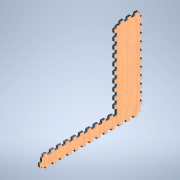
# Autodesk Inventor part: plate_side
Saved by Autodesk Inventor 2021 (Build 250183000, 183)
## iProperties
Created: 2021-03-07
Part Number: plate_side
Material: Generisch
Document SubType Name: Modeling
Designer: Tilman
Density: 1 g/cm^3
Appearance: Glänzend - Schwarz
Author: Tilman
Autodesk Inventor part; units mm, degrees
ref_plane "YZ Plane" through (0, 0, 0) normal (1, 0, 0) x (0, 1, 0)
ref_plane "XZ Plane" through (0, 0, 0) normal (0, 1, 0) x (-1, 0, 0)
ref_plane "XY Plane" through (0, 0, 0) normal (0, 0, 1) x (1, 0, 0)
sketch "Skizze1" plane through (0, 0, 0) normal (1, 0, 0) x (0, 1, 0)
  line L0 (5, 0) -> (5, -3)
  line L1 (5, -3) -> (3, -3)
  line L2 (3, -3) -> (3, -8)
  line L3 (3, -8) -> (0, -8)
  line L4 (0, -8) -> (0, -13)
  line L5 (0, -13) -> (3, -13)
  line L6 (3, -13) -> (3, -18)
  line L7 (3, -18) -> (0, -18)
  line L8 (0, -18) -> (0, -23)
  line L9 (0, -23) -> (3, -23)
  line L10 (3, -23) -> (3, -28)
  line L11 (3, -28) -> (0, -28)
  line L12 (0, -28) -> (0, -33)
  line L13 (0, -33) -> (3, -33)
  line L14 (3, -33) -> (3, -38)
  line L15 (3, -38) -> (0, -38)
  line L16 (0, -38) -> (0, -43)
  line L17 (0, -43) -> (3, -43)
  line L18 (3, -43) -> (3, -48)
  line L19 (3, -48) -> (0, -48)
  line L20 (0, -48) -> (0, -53)
  line L21 (0, -53) -> (3, -53)
  line L22 (3, -53) -> (3, -58)
  line L23 (3, -58) -> (0, -58)
  line L24 (0, -58) -> (0, -63)
  line L25 (0, -63) -> (3, -63)
  line L26 (3, -63) -> (3, -68)
  line L27 (3, -68) -> (0, -68)
  line L28 (0, -68) -> (0, -73)
  line L29 (0, -73) -> (3, -73)
  line L30 (3, -73) -> (3, -78)
  line L31 (3, -78) -> (0, -78)
  line L32 (0, -78) -> (0, -83)
  line L33 (0, -83) -> (3, -83)
  line L34 (3, -83) -> (3, -88)
  line L35 (3, -88) -> (0, -88)
  line L36 (0, -88) -> (0, -93)
  line L37 (0, -93) -> (3, -93)
  line L38 (3, -93) -> (3, -98)
  line L39 (3, -98) -> (0, -98)
  line L40 (0, -98) -> (0, -103)
  line L41 (0, -103) -> (3, -103)
  line L42 (3, -133) -> (3, -137)
  line L43 (3, -137) -> (10, -137)
  line L44 (10, -137) -> (10, -140)
  line L45 (10, -140) -> (15, -140)
  line L46 (15, -140) -> (15, -137)
  line L47 (15, -137) -> (20, -137)
  line L48 (25, -137) -> (30, -137)
  line L49 (25, -140) -> (25, -137)
  line L50 (20, -140) -> (25, -140)
  line L51 (20, -137) -> (20, -140)
  line L52 (35, -137) -> (40, -137)
  line L53 (35, -140) -> (35, -137)
  line L54 (30, -140) -> (35, -140)
  line L55 (30, -137) -> (30, -140)
  line L56 (45, -137) -> (50, -137)
  line L57 (45, -140) -> (45, -137)
  line L58 (40, -140) -> (45, -140)
  line L59 (40, -137) -> (40, -140)
  line L60 (55, -137) -> (60, -137)
  line L61 (55, -140) -> (55, -137)
  line L62 (50, -140) -> (55, -140)
  line L63 (50, -137) -> (50, -140)
  line L64 (65, -137) -> (70, -137)
  line L65 (65, -140) -> (65, -137)
  line L66 (60, -140) -> (65, -140)
  line L67 (60, -137) -> (60, -140)
  line L68 (75, -137) -> (80, -137)
  line L69 (75, -140) -> (75, -137)
  line L70 (70, -140) -> (75, -140)
  line L71 (70, -137) -> (70, -140)
  line L72 (85, -137) -> (90, -137)
  line L73 (85, -140) -> (85, -137)
  line L74 (80, -140) -> (85, -140)
  line L75 (80, -137) -> (80, -140)
  line L76 (95, -137) -> (100, -137)
  line L77 (95, -140) -> (95, -137)
  line L78 (90, -140) -> (95, -140)
  line L79 (90, -137) -> (90, -140)
  line L80 (105, -137) -> (110, -137)
  line L81 (105, -140) -> (105, -137)
  line L82 (100, -140) -> (105, -140)
  line L83 (100, -137) -> (100, -140)
  line L84 (115, -137) -> (120, -137)
  line L85 (115, -140) -> (115, -137)
  line L86 (110, -140) -> (115, -140)
  line L87 (110, -137) -> (110, -140)
  line L88 (120, -137) -> (120, -135)
  line L89 (120, -135) -> (123, -135)
  line L90 (123, -135) -> (123, -130)
  line L91 (123, -130) -> (120, -130)
  line L92 (120, -130) -> (120, -125)
  line L93 (120, -105) -> (118, -105)
  line L94 (118, -105) -> (118, -102)
  line L95 (118, -102) -> (113, -102)
  line L96 (113, -102) -> (113, -105)
  line L97 (113, -105) -> (108, -105)
  line L98 (103, -105) -> (98, -105)
  line L99 (103, -102) -> (103, -105)
  line L100 (108, -102) -> (103, -102)
  line L101 (108, -105) -> (108, -102)
  line L102 (93, -105) -> (88, -105)
  line L103 (93, -102) -> (93, -105)
  line L104 (98, -102) -> (93, -102)
  line L105 (98, -105) -> (98, -102)
  line L106 (83, -105) -> (78, -105)
  line L107 (83, -102) -> (83, -105)
  line L108 (88, -102) -> (83, -102)
  line L109 (88, -105) -> (88, -102)
  line L110 (73, -105) -> (68, -105)
  line L111 (73, -102) -> (73, -105)
  line L112 (78, -102) -> (73, -102)
  line L113 (78, -105) -> (78, -102)
  line L114 (63, -105) -> (58, -105)
  line L115 (63, -102) -> (63, -105)
  line L116 (68, -102) -> (63, -102)
  line L117 (68, -105) -> (68, -102)
  line L118 (53, -105) -> (48, -105)
  line L119 (53, -102) -> (53, -105)
  line L120 (58, -102) -> (53, -102)
  line L121 (58, -105) -> (58, -102)
  line L122 (43, -105) -> (38, -105)
  line L123 (43, -102) -> (43, -105)
  line L124 (48, -102) -> (43, -102)
  line L125 (48, -105) -> (48, -102)
  line L126 (33, -105) -> (28, -105)
  line L127 (33, -102) -> (33, -105)
  line L128 (38, -102) -> (33, -102)
  line L129 (38, -105) -> (38, -102)
  line L130 (23, -105) -> (18, -105)
  line L131 (23, -102) -> (23, -105)
  line L132 (28, -102) -> (23, -102)
  line L133 (28, -105) -> (28, -102)
  line L134 (5, 0) -> (10, 0)
  line L135 (10, 0) -> (10, -3)
  line L136 (10, -3) -> (15, -3)
  line L137 (18, -105) -> (15, -105)
  line L138 (15, -105) -> (15, -100)
  line L139 (15, -100) -> (18, -100)
  line L140 (18, -100) -> (18, -95)
  line L141 (18, -90) -> (18, -85)
  line L142 (18, -95) -> (15, -95)
  line L143 (15, -90) -> (18, -90)
  line L144 (15, -95) -> (15, -90)
  line L145 (18, -80) -> (18, -75)
  line L146 (18, -85) -> (15, -85)
  line L147 (15, -80) -> (18, -80)
  line L148 (15, -85) -> (15, -80)
  line L149 (18, -70) -> (18, -65)
  line L150 (18, -75) -> (15, -75)
  line L151 (15, -70) -> (18, -70)
  line L152 (15, -75) -> (15, -70)
  line L153 (18, -60) -> (18, -55)
  line L154 (18, -65) -> (15, -65)
  line L155 (15, -60) -> (18, -60)
  line L156 (15, -65) -> (15, -60)
  line L157 (18, -50) -> (18, -45)
  line L158 (18, -55) -> (15, -55)
  line L159 (15, -50) -> (18, -50)
  line L160 (15, -55) -> (15, -50)
  line L161 (18, -40) -> (18, -35)
  line L162 (18, -45) -> (15, -45)
  line L163 (15, -40) -> (18, -40)
  line L164 (15, -45) -> (15, -40)
  line L165 (18, -30) -> (18, -25)
  line L166 (18, -35) -> (15, -35)
  line L167 (15, -30) -> (18, -30)
  line L168 (15, -35) -> (15, -30)
  line L169 (3, -103) -> (3, -108)
  line L170 (3, -108) -> (0, -108)
  line L171 (0, -108) -> (0, -113)
  line L172 (0, -113) -> (3, -113)
  line L173 (3, -113) -> (3, -118)
  line L174 (3, -118) -> (0, -118)
  line L175 (0, -118) -> (0, -123)
  line L176 (0, -123) -> (3, -123)
  line L177 (18, -20) -> (18, -15)
  line L178 (18, -25) -> (15, -25)
  line L179 (15, -20) -> (18, -20)
  line L180 (15, -25) -> (15, -20)
  line L181 (18, -10) -> (18, -5)
  line L182 (18, -15) -> (15, -15)
  line L183 (15, -10) -> (18, -10)
  line L184 (15, -15) -> (15, -10)
  line L185 (15, -5) -> (18, -5)
  line L186 (3, -123) -> (3, -128)
  line L187 (3, -128) -> (0, -128)
  line L188 (0, -128) -> (0, -133)
  line L189 (0, -133) -> (3, -133)
  line L190 (15, -5) -> (15, -3)
  line L191 (120, -120) -> (120, -115)
  line L192 (120, -125) -> (123, -125)
  line L193 (123, -120) -> (120, -120)
  line L194 (123, -125) -> (123, -120)
  line L195 (120, -110) -> (120, -105)
  line L196 (120, -115) -> (123, -115)
  line L197 (123, -110) -> (120, -110)
  line L198 (123, -115) -> (123, -110)
  point P0 (0, 0)
  point P1 (108, -105)
  point P2 (98, -105)
  point P3 (88, -105)
  point P4 (78, -105)
  point P5 (68, -105)
  point P6 (58, -105)
  point P7 (48, -105)
  point P8 (38, -105)
  point P9 (28, -105)
  dimension "d0" = 3
  dimension "d1" = 5
  dimension "d2" = 2
  dimension "d5" = 10
  dimension "d10" = 4
  dimension "d11" = 7
  dimension "d14" = 10
  dimension "d28" = 10
  dimension "d35" = 10
  dimension "d44" = 10
  constraints: 398 end point, 21 equal length, 20 perpendicular, 17 point on line, 7 vertical, 6 horizontal, 4 collinear, 2 coincident, 2 vertical alignment, 1 horizontal alignment, 374 other
  measures "d0" distance of L2.end L3.end
  measures "d1" distance of L3.end L4.end
  measures "d2" distance of L0.end L1.end
  measures "d5" distance of L2.end L6.end
  measures "d10" distance of L42.start L42.end
  measures "d11" distance of L42.end L43.end
  measures "d14" distance of L46.end L48.start
  measures "d28" distance of L97.end L98.end
  measures "d35" distance of L138.end L143.start
  measures "d44" distance of L88.end L192.start
extrude "Extrusion1" add sketch "Skizze1" along normal blind 3
